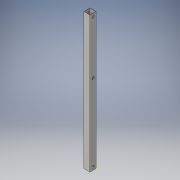
# Autodesk Inventor part: 1x1 16th Inch Aluminum Tube - Custom for Lift Arms
Saved by Autodesk Inventor 2016 (Build 200138000, 138)
## iProperties
Created: 2016-01-28
Part Number: 1x1 16th Inch Aluminum Tube - Custom for Lift Arms
Material: Generic
Document SubType Name: Modeling
Designer: Jack Jaworski
Density: 1 g/cm^3
Appearance: Default
Author: Jack Jaworski
Autodesk Inventor part; units mm, degrees
ref_plane "YZ Plane" through (0, 0, 0) normal (1, 0, 0) x (0, 1, 0)
ref_plane "XZ Plane" through (0, 0, 0) normal (0, 1, 0) x (-1, 0, 0)
ref_plane "XY Plane" through (0, 0, 0) normal (0, 0, 1) x (1, 0, 0)
sketch "Sketch1" plane through (0, 0, 0) normal (0, 1, 0) x (-1, 0, 0)
  line L0 (0, 0) -> (25.4, 0)
  line L1 (25.4, 0) -> (25.4, 25.4)
  line L2 (25.4, 25.4) -> (0, 25.4)
  line L3 (0, 25.4) -> (0, 0)
  line L4 (23.8125, 23.8125) -> (1.5875, 23.8125)
  line L5 (1.5875, 23.8125) -> (1.5875, 1.5875)
  line L6 (1.5875, 1.5875) -> (23.8125, 1.5875)
  line L7 (23.8125, 1.5875) -> (23.8125, 23.8125)
  dimension "d0" = 25.4
  dimension "d1" = 25.4
  dimension "d2" = 1.5875
  dimension "d3" = 1.5875
  dimension "d4" = 1.5875
  dimension "d5" = 1.5875
  constraints: 16 end point, 4 parallel, 2 horizontal, 2 perpendicular
  measures "d0" distance of L1.end L2.end
  measures "d1" distance of L0.end L1.end
  measures "d2" distance between parallel lines of L1 L7
  measures "d3" distance between parallel lines of L0 L6
  measures "d4" distance between parallel lines of L2 L4
  measures "d5" distance between parallel lines of L3 L5
extrude "Extrusion1" add sketch "Sketch1" along normal blind 548.64
sketch "Sketch2" plane through (0, 0, 25.4) normal (1, 0, 0) x (0, 0, -1)
  circle A0 centre (12.7, 12.7) radius 5.08
  line L0 (25.4, 0) -> (25.4, 548.64) projected
  line L1 (0, 0) -> (25.4, 0) projected
  dimension "d9" = 12.7
  dimension "d10" = 10.16
  dimension "d11" = 12.7
  constraints: 1 centre point
  measures "d9" distance from line of L0 A0.centre
  measures "d10" diameter of A0
  measures "d11" distance from line of L1 A0.centre
extrude "Extrusion2" cut sketch "Sketch2" against normal blind 25.4
sketch "Sketch3" plane through (0, 0, 25.4) normal (1, 0, 0) x (0, 0, -1)
  circle A0 centre (12.7, 535.94) radius 5.08
  line L0 (25.4, 0) -> (25.4, 548.64) projected
  line L1 (0, 548.64) -> (25.4, 548.64) projected
  dimension "d14" = 12.7
  dimension "d15" = 12.7
  dimension "d16" = 10.16
  constraints: 1 centre point
  measures "d14" distance from line of L0 A0.centre
  measures "d15" distance from line of A0.centre L1
  measures "d16" diameter of A0
extrude "Extrusion3" cut sketch "Sketch3" against normal blind 25.4
sketch "Sketch4" plane through (0, 0, 25.4) normal (1, 0, 0) x (0, 0, -1)
  point P0 (25.4, 0)
sketch "Sketch5" plane through (0, 0, 25.4) normal (1, 0, 0) x (0, 0, -1)
  circle A0 centre (12.7, 322.58) radius 5.08
  line L0 (0, 0) -> (0, 548.64) projected
  circle A1 centre (12.7, 535.94) radius 5.08 projected
  point P0 (25.4, 0)
  dimension "d19" = 10.16
  dimension "d20" = 12.7
  dimension "d21" = 213.36
  constraints: 1 centre point
  measures "d19" diameter of A0
  measures "d20" distance from line of L0 A0.centre
  measures "d21" distance of A0.centre A1.centre
extrude "Extrusion4" cut sketch "Sketch5" against normal blind 25.4 contours A0
body "Solid1"
